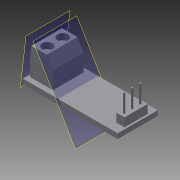
# Autodesk Inventor part: ACS712(prudovy snimac)
Saved by Autodesk Inventor 2015 (Build 190159000, 159)
## iProperties
Created: 2015-11-17
Part Number: ACS712(prudovy snimac)
Material: Generic
Document SubType Name: Modeling
Designer: Jufo
Density: 1 g/cm^3
Appearance: Default
Author: Jufo
Autodesk Inventor part; units mm, degrees
ref_plane "YZ Plane" through (0, 0, 0) normal (1, 0, 0) x (0, 1, 0)
ref_plane "XZ Plane" through (0, 0, 0) normal (0, 1, 0) x (-1, 0, 0)
ref_plane "XY Plane" through (0, 0, 0) normal (0, 0, 1) x (1, 0, 0)
sketch "Sketch1" plane through (0, 0, 0) normal (0, 1, 0) x (-1, 0, 0)
  line L0 (25.0064, 9.2593) -> (-5.9936, 9.2593)
  line L1 (-5.9936, 9.2593) -> (-5.9936, -3.7407)
  line L2 (-5.9936, -3.7407) -> (25.0064, -3.7407)
  line L3 (25.0064, -3.7407) -> (25.0064, 9.2593)
  point P0 (0, 0)
  dimension "d0" = 31
  dimension "d1" = 13
  constraints: 8 end point, 2 parallel, 1 horizontal, 1 perpendicular
  measures "d0" distance of L2.end L1.end
  measures "d1" distance of L1.end L0.end
extrude "Extrusion1" add sketch "Sketch1" along normal blind 1.6
sketch "Sketch2" plane through (0, 1.6, 0) normal (0, 1, 0) x (1, 0, 0)
  line L0 (5.9936, -9.2593) -> (5.9936, 3.7407) projected
  line L1 (5.9936, 3.7407) -> (-25.0064, 3.7407) projected
  line L2 (5.3936, -6.4593) -> (5.3936, 1.1407)
  line L3 (5.3936, 1.1407) -> (2.7936, 1.1407)
  line L4 (2.7936, 1.1407) -> (2.7936, -6.4593)
  line L5 (2.7936, -6.4593) -> (5.3936, -6.4593)
  point P0 (0, 0)
  point P1 (5.9936, 1.1407)
  point P2 (5.9936, -6.4593)
  dimension "d9" = 2.6
  dimension "d10" = 7.6
  dimension "d12" = 2.6
  dimension "d13" = 0.6
  constraints: 8 end point, 3 perpendicular, 2 point on line, 1 vertical
  measures "d9" distance of L2.end L3.end
  measures "d10" distance of L3.end L4.end
  measures "d12" distance between parallel lines of L1 L3
  measures "d13" distance between parallel lines of L0 L2
extrude "Extrusion2" add sketch "Sketch2" along normal blind 2.8
sketch "Sketch3" plane through (0, 4.4, 0) normal (0, 1, 0) x (1, 0, 0)
  circle A0 centre (4.0936, -5.2593) radius 0.3
  circle A1 centre (4.0936, -2.6593) radius 0.3
  circle A2 centre (4.0936, -0.0593) radius 0.3
  line L0 (5.3936, -6.4593) -> (5.3936, 1.1407) projected
  line L1 (2.7936, -6.4593) -> (5.3936, -6.4593) projected
  point P0 (0, 0)
  dimension "d14" = 0.6
  dimension "d15" = 0.6
  dimension "d16" = 0.6
  dimension "d17" = 1.3
  dimension "d18" = 1.3
  dimension "d19" = 1.3
  dimension "d20" = 2
  dimension "d21" = 2
  dimension "d22" = 1.2
  constraints: 3 centre point
  measures "d14" diameter of A0
  measures "d15" diameter of A1
  measures "d16" diameter of A2
  measures "d17" distance from line of L0 A0.centre
  measures "d18" distance from line of L0 A1.centre
  measures "d19" distance from line of L0 A2.centre
  measures "d22" distance from line of L1 A0.centre
extrude "Extrusion3" add sketch "Sketch3" along normal blind 5.8
sketch "Sketch4" plane through (0, 1.6, 0) normal (0, 1, 0) x (1, 0, 0)
  line L0 (-24.1064, -7.6593) -> (-16.7064, -7.6593)
  line L1 (-16.7064, -7.6593) -> (-16.7064, 2.3407)
  line L2 (-16.7064, 2.3407) -> (-24.1064, 2.3407)
  line L3 (-24.1064, 2.3407) -> (-24.1064, -7.6593)
  line L4 (-25.0064, 3.7407) -> (-25.0064, -9.2593) projected
  line L5 (-25.0064, -9.2593) -> (5.9936, -9.2593) projected
  point P0 (0, 0)
  dimension "d25" = 7.4
  dimension "d26" = 10
  dimension "d27" = 0.9
  dimension "d28" = 1.6
  constraints: 8 end point, 2 parallel, 1 horizontal, 1 perpendicular
  measures "d25" distance of L2.end L1.end
  measures "d26" distance of L1.end L0.end
  measures "d27" distance between parallel lines of L4 L3
  measures "d28" distance between parallel lines of L5 L0
extrude "Extrusion4" add sketch "Sketch4" along normal blind 5.6
sketch "Sketch5" plane through (0, 7.2, 0) normal (0, 1, 0) x (1, 0, 0)
  line L0 (-23.7064, -7.6593) -> (-18.7064, -7.6593)
  line L1 (-18.7064, -7.6593) -> (-18.7064, 2.3407)
  line L2 (-18.7064, 2.3407) -> (-23.7064, 2.3407)
  line L3 (-23.7064, 2.3407) -> (-23.7064, -7.6593)
  line L4 (-24.1064, -7.6593) -> (-16.7064, -7.6593) projected
  line L5 (-24.1064, 2.3407) -> (-16.7064, 2.3407) projected
  line L6 (-16.7064, -7.6593) -> (-16.7064, 2.3407) projected
  point P0 (0, 0)
  dimension "d31" = 5
  dimension "d32" = 0
  dimension "d33" = 0
  dimension "d34" = 2
  constraints: 8 end point, 3 perpendicular, 1 horizontal
  measures "d31" distance of L0.start L0.end
  measures "d32" distance between parallel lines of L0 L4
  measures "d33" distance between parallel lines of L5 L2
  measures "d34" distance between parallel lines of L6 L1
extrude "Extrusion5" add sketch "Sketch5" along normal blind 3.4 contours L3 L2 L1 L0
ref_plane "Work Plane1" through (-24.1064, 7.2, -2.3407) normal (-0.9931506, 0.1168412, 0) x (0, 0, 1)
sketch "Sketch6" plane through (-24.1064, 7.2, -2.3407) normal (-0.9931506, 0.1168412, 0) x (0, 0, 1)
  line L0 (0, 3.4234) -> (0, 0)
  line L1 (0, 0) -> (10, 0) projected
  line L2 (0, 0) -> (10, 0)
  line L3 (10, 0) -> (10, 3.4234)
  line L4 (10, 3.4234) -> (0, 3.4234)
  line L5 (0, 3.4234) -> (10, 3.4234) projected
  point P0 (2.3407, -4.3341)
  constraints: 8 end point, 3 perpendicular, 1 collinear
extrude "Extrusion6" add sketch "Sketch6" against normal blind 1
ref_plane "Work Plane2" through (-18.7064, 10.6, 7.6593) normal (-0.8619342, -0.5070201, 0) x (0, 0, -1)
sketch "Sketch7" plane through (-18.7064, 10.6, 7.6593) normal (-0.8619342, -0.5070201, 0) x (0, 0, -1)
  line L0 (0, 0) -> (0, 3.9446)
  line L1 (0, 3.9446) -> (10, 3.9446)
  line L2 (0, 3.9446) -> (10, 3.9446) projected
  line L3 (10, 3.9446) -> (10, 0)
  line L4 (10, 0) -> (0, 0)
  point P0 (7.6593, 18.621)
  constraints: 8 end point, 2 perpendicular, 1 collinear, 1 vertical
extrude "Extrusion7" add sketch "Sketch7" along normal blind 2
sketch "Sketch8" plane through (0, 10.6, 0) normal (0, 1, 0) x (1, 0, 0)
  circle A0 centre (-21.0064, -0.1593) radius 1.7
  circle A1 centre (-21.0064, -5.1593) radius 1.7
  line L0 (-18.7064, 2.3407) -> (-23.7064, 2.3407) projected
  line L1 (-23.7064, 2.3407) -> (-23.7064, -7.6593) projected
  point P0 (0, 0)
  dimension "d41" = 3.4
  dimension "d42" = 3.4
  dimension "d43" = 2.5
  dimension "d44" = 5
  dimension "d45" = 2.7
  dimension "d46" = 2.7
  constraints: 2 centre point
  measures "d41" diameter of A0
  measures "d42" diameter of A1
  measures "d43" distance from line of L0 A0.centre
  measures "d44" distance of A0.centre A1.centre
  measures "d45" distance from line of A1.centre L1
  measures "d46" distance from line of L1 A0.centre
extrude "Extrusion8" cut sketch "Sketch8" against normal blind 2
sketch "Sketch9" plane through (0, 1.6, 0) normal (0, 1, 0) x (1, 0, 0)
  line L0 (-14.7064, -5.2593) -> (-10.7064, -5.2593)
  line L1 (-10.7064, -5.2593) -> (-10.7064, -0.2593)
  line L2 (-10.7064, -0.2593) -> (-14.7064, -0.2593)
  line L3 (-14.7064, -0.2593) -> (-14.7064, -5.2593)
  line L4 (-16.7064, -7.6593) -> (-16.7064, 2.3407) projected
  line L5 (5.9936, 3.7407) -> (-25.0064, 3.7407) projected
  point P0 (0, 0)
  dimension "d49" = 4
  dimension "d50" = 5
  dimension "d51" = 2
  dimension "d52" = 4
  constraints: 8 end point, 2 parallel, 1 horizontal, 1 perpendicular
  measures "d49" distance of L2.end L1.end
  measures "d50" distance of L1.end L0.end
  measures "d51" distance between parallel lines of L4 L3
  measures "d52" distance between parallel lines of L5 L2
extrude "Extrusion9" add sketch "Sketch9" along normal blind 1.4
fillet "Fillet1" radius 0.2 4 edges at (-10.7064, 3, 2.7593) (-12.7064, 3, 5.2593) (-14.7064, 3, 2.7593) (-12.7064, 3, 0.2593)
equation "\"d18\" = d17"
equation "\"d19\" = d17"
equation "\"d46\" = d45"
body "Solid1"
